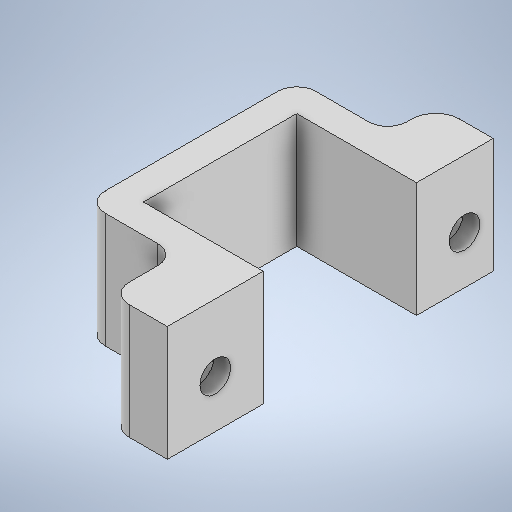
# Autodesk Inventor part: motorMount
Saved by Autodesk Inventor 2025.1 (Build 291241020, 241B)
## iProperties
Created: 2022-06-21
Part Number: motorMount
Material: Generic
Document SubType Name: Modeling
Designer: scottst
Density: 1 g/cm^3
Appearance: Default
Author: scottst
Autodesk Inventor part; units mm, degrees
sketch "Sketch1" plane through (0, 0, 0) normal (0, 1, 0) x (-1, 0, 0)
  line L0 (-6, 8) -> (4.5, 8)
  line L1 (4.5, 8) -> (4.5, -8)
  line L2 (4.5, -8) -> (-6, -8)
  line L3 (-6, 11) -> (7.5, 11)
  line L4 (7.5, 11) -> (7.5, -11)
  line L5 (7.5, -11) -> (-6, -11)
  line L6 (-6, -8) -> (-6, -11)
  line L7 (-6, 8) -> (-6, 11)
  line L8 (-6, -8) -> (-6, -18)
  line L9 (-6, 8) -> (-6, 18)
  line L10 (-6, 18) -> (0, 18)
  line L11 (0, 18) -> (0, 11)
  line L12 (-6, -18) -> (0, -18)
  line L13 (0, -18) -> (0, -11)
  line L14 (4.5, 0) -> (1.2283, 0)
  line L15 (7.5, 0) -> (11.9514, 0)
  dimension "d0" = 10.5
  dimension "d1" = 16
  dimension "d3" = 22
  dimension "d4" = 3
  dimension "d5" = 10
  dimension "d6" = 10
  dimension "d7" = 6
  dimension "d8" = 6
  dimension "d30" = 10.5
  constraints: 32 end point, 6 perpendicular, 5 horizontal, 3 point on line, 2 midpoint, 2 parallel, 1 vertical, 2 other
  measures "d0" distance of L1.end L2.end
  measures "d1" distance of L0.end L1.end
  measures "d3" distance of L3.end L4.end
  measures "d4" distance of L3.start L0.start
  measures "d5" distance of L2.end L8.end
  measures "d6" distance of L0.start L9.end
  measures "d7" distance of L9.end L10.end
  measures "d8" distance of L8.end L12.end
  measures "d30" distance of L0.start L0.end
extrude "Extrusion1" add sketch "Sketch1" along normal blind 14
ref_plane "Work Plane1" through (3.5, 0, 18) normal (1, 0, 0) x (0, 0, -1)
sketch "Sketch2" plane through (3.5, 0, 18) normal (1, 0, 0) x (0, 0, -1)
  line L0 (0, 14) -> (10, 14) construction
  line L1 (0, 0) -> (10, 14) construction
  line L2 (10, 14) -> (0, 14) construction
  line L3 (0, 0) -> (10, 0) construction
  line L4 (0, 14) -> (10, 0) construction
  circle A0 centre (5, 7) radius 1.6
  line L5 (5, 7) -> (7, 4.9696) construction
  line L6 (7, 0) -> (7, 14) construction
  line L7 (5, 7) -> (7.85, 7) construction
  line L8 (7.85, 5.3546) -> (5, 3.7091)
  line L9 (5, 3.7091) -> (2.15, 5.3546)
  line L10 (2.15, 5.3546) -> (2.15, 8.6454)
  line L11 (2.15, 8.6454) -> (5, 10.2909)
  line L12 (5, 10.2909) -> (7.85, 8.6454)
  line L13 (7.85, 8.6454) -> (7.85, 5.3546)
  line L14 (10, 14) -> (26, 14) projected
  line L15 (18, 14) -> (18, 5.4848)
  point P0 (18, 0)
  dimension "d12" = 3.2
  dimension "d13" = 2.85
  dimension "d14" = 2.85
  constraints: 24 end point, 3 midpoint, 1 centre point, 1 coincident, 1 collinear, 1 horizontal, 1 point on line, 1 vertical, 13 other
  measures "d12" diameter of A0
  measures "d13" distance of L5.start L5.end
  measures "d14" distance of L5.start L7.end
extrude "Extrusion2" cut sketch "Sketch2" along normal blind 15 and the other way blind 3.8 contours A0
extrude "Extrusion3" cut sketch "Sketch2" along normal blind 0.75 and the other way blind 1.75
ref_plane "Work Plane2" through (6, 0, 0) normal (0, 0, -1) x (-1, 0, 0)
mirror "Mirror1" about plane through (6, 0, 0) normal (0, 0, -1) of "Extrusion2", "Extrusion3"
sketch "Sketch3" plane through (3.5, 0, 18) normal (1, 0, 0) x (0, 0, -1)
  line L0 (31, 10.2909) -> (28.15, 8.6454) projected
  line L1 (28.15, 8.6454) -> (28.15, 10.2835)
  line L2 (33.85, 5.3546) -> (33.85, 8.6454) projected
  line L3 (33.85, 8.6454) -> (33.85, 10.2835)
  line L4 (33.85, 10.2835) -> (28.15, 10.2835)
  line L5 (28.15, 8.6454) -> (33.85, 8.6454)
  line L6 (7.85, 8.6454) -> (7.85, 5.3546) projected
  line L7 (7.85, 8.6454) -> (7.85, 10.2835)
  line L8 (7.85, 10.2835) -> (2.1555, 10.2835)
  line L9 (2.1555, 10.2835) -> (2.1555, 8.6454)
  line L10 (5, 10.2909) -> (7.85, 8.6454) projected
  line L11 (2.1555, 8.6454) -> (7.85, 8.6454)
  line L12 (2.15, 5.3546) -> (2.15, 8.6454) projected
  point P0 (18, 0)
  point P1 (7.85, 7)
  dimension "d24" = 5.7
  constraints: 16 end point, 4 perpendicular, 3 vertical, 1 midpoint, 1 parallel
  measures "d24" distance from line of L12 point (7.85, 7)
extrude "Extrusion4" cut sketch "Sketch3" along normal blind 0.75 and the other way blind 1.75
ref_plane "Work Plane4" through (-4.5, 0, 8) normal (1, 0, 0) x (0, 0, -1)
split body "Split1" result two bodies by plane through (-4.5, 0, 8) normal (1, 0, 0) first body at (2.5, 4.6667, 8.5) (-1, 4.6667, -8.5)
move or copy body "Move Body1" bodies to move or copy 2 copy no translate (2, 0, 0)
sketch "Sketch4" plane through (-2.5, 0, 8) normal (-1, 0, 0) x (0, 0, 1)
  line L0 (3, 0) -> (5, 0) projected
  line L1 (3, 0) -> (0, 0)
  line L2 (0, 0) -> (0, 14)
  line L3 (0, 14) -> (3, 14)
  line L4 (3, 14) -> (3, 0)
  line L5 (-16, 0) -> (-16, 14) projected
  line L6 (-19, 0) -> (-19, 14) projected
  line L7 (-16, 0) -> (-19, 0)
  line L8 (-19, 0) -> (-19, 14)
  line L9 (-19, 14) -> (-16, 14)
  line L10 (-16, 14) -> (-16, 0)
  point P0 (-8, 0)
  constraints: 16 end point, 4 parallel, 2 horizontal, 2 perpendicular
extrude "Extrusion5" add sketch "Sketch4" along normal up to surface (2 mm away) bodies 2
combine bodies "Combine1" operation type add bodies to combine 3 2
fillet "Fillet3" radius 2 6 edges at (-7.5, 7, 11) (2, 7, 18) (-7.5, 7, -11) (2, 7, -18) (2, 7, -11) (2, 7, 11)
sketch "Sketch5" plane through (-4.5, 14, 8) normal (0, 1, 0) x (1, 0, 0)
  line L0 (6.5, 24) -> (6.5, 21) projected
  line L1 (12.5, 26) -> (6.5, 26)
  line L2 (6.5, 26) -> (6.5, 24)
  line L3 (6.5, 24) -> (12.5, 24)
  line L4 (12.5, 24) -> (12.5, 26)
  point P0 (4.5, 8)
  constraints: 8 end point, 2 parallel, 1 horizontal, 1 perpendicular
extrude "Extrusion6" cut sketch "Sketch5" against normal blind 18 bodies 3
sketch "Sketch6" plane through (-7.5, 0, -9) normal (-1, 0, 0) x (0, 0, 1)
  line L0 (-7, 0) -> (-4, 0) projected
  line L1 (27, 0) -> (27, 14) projected
  line L2 (-7, 0) -> (27, 0)
  line L3 (27, 0) -> (27, 2)
  line L4 (27, 2) -> (-7, 2)
  line L5 (-7, 2) -> (-7, 0)
  point P0 (9, 0)
  dimension "d40" = 2
  constraints: 8 end point, 2 parallel, 1 horizontal, 1 perpendicular, 1 point on line
  measures "d40" distance of L3.end L2.end
extrude "Extrusion7" cut sketch "Sketch6" against normal blind 18 bodies 3
fillet "Fillet4" radius 2.5 1 edges at (2, 8, -16)
ref_plane "Work Plane3" through (6, 0, 0) normal (0, 0, -1) x (-1, 0, 0)
body "Solid3"
